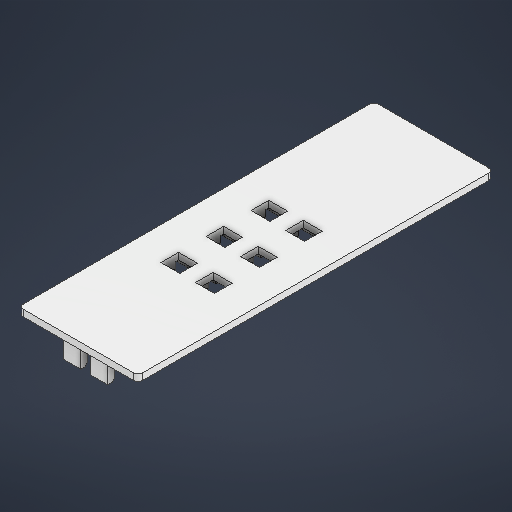
# Autodesk Inventor part: module-lid_switch
Saved by Autodesk Inventor 2025.4 (Build 294407000, 407)
## iProperties
Created: 2025-09-07
Part Number: module-lid_switch
Material: PC/ABS Plastic
Document SubType Name: Modeling
Designer: sam
Density: 1.1 g/cm^3
Appearance: Smooth - White
Author: sam
Autodesk Inventor part; units mm, degrees
ref_plane "YZ Plane" through (0, 0, 0) normal (1, 0, 0) x (0, 1, 0)
ref_plane "XZ Plane" through (0, 0, 0) normal (0, 1, 0) x (-1, 0, 0)
ref_plane "XY Plane" through (0, 0, 0) normal (0, 0, 1) x (1, 0, 0)
sketch "Sketch1" plane through (0, 0, 0) normal (0, 1, 0) x (-1, 0, 0)
  line L0 (-27.2, -81) -> (27.2, -81)
  line L1 (27.2, -81) -> (27.2, 81)
  line L2 (27.2, 81) -> (-27.2, 81)
  line L3 (-27.2, 81) -> (-27.2, -81)
  line L4 (-27.2, -81) -> (27.2, 81) construction
  line L5 (27.2, -81) -> (-27.2, 81) construction
  point P0 (0, 0)
  dimension "d0" = 54.4
  dimension "d1" = 162
  constraints: 12 end point, 2 midpoint, 2 parallel, 1 horizontal, 1 perpendicular
  measures "d0" distance of L2.end L1.end
  measures "d1" distance between parallel lines of L0 L2
extrude "Extrusion1" add sketch "Sketch1" along normal blind 3
sketch "Sketch2" plane through (0, 0, 0) normal (0, -1, 0) x (1, 0, 0)
  line L0 (24, 77.8) -> (-24, 77.8)
  line L1 (-24, 77.8) -> (-24, -77.8)
  line L2 (-24, -77.8) -> (24, -77.8)
  line L3 (24, -77.8) -> (24, 77.8)
  line L4 (24, 77.8) -> (-24, -77.8) construction
  line L5 (-24, 77.8) -> (24, -77.8) construction
  line L6 (-27.2, -81) -> (-27.2, 81) projected
  line L7 (27.2, -81) -> (-27.2, -81) projected
  point P0 (0, 0)
  dimension "d4" = 3.2
  dimension "d5" = 3.2
  constraints: 12 end point, 2 midpoint, 2 parallel, 1 horizontal, 1 perpendicular
  measures "d4" distance between parallel lines of L6 L1
  measures "d5" distance between parallel lines of L7 L2
extrude "Extrusion2" add sketch "Sketch2" along normal blind 3
fillet "Fillet1" radius 2 8 edges at (27.2, 1.5, 81) (24, -1.5, 77.8) (-24, -1.5, 77.8) (-27.2, 1.5, 81) (24, -1.5, -77.8) (27.2, 1.5, -81) (-27.2, 1.5, -81) (-24, -1.5, -77.8)
fillet "Fillet2" radius 0.5 8 edges at (-23.4142, -3, 77.2142) (-24, -3, 0) (-23.4142, -3, -77.2142) (0, -3, -77.8) (23.4142, -3, -77.2142) (24, -3, 0) (23.4142, -3, 77.2142) (0, -3, 77.8)
sketch "Sketch3" plane through (0, -3, 0) normal (0, -1, 0) x (1, 0, 0)
  line L0 (-22, 77.8) -> (22, 77.8) projected
  line L1 (-10.2, 77.8) -> (-2.14, 77.8)
  line L2 (-2.14, 77.8) -> (-2.14, 74.8)
  line L3 (-2.14, 74.8) -> (-10.2, 74.8)
  line L4 (-10.2, 74.8) -> (-10.2, 77.8)
  line L5 (-27.2, -79) -> (-27.2, 79) projected
  line L6 (2.14, 77.8) -> (10.2, 77.8)
  line L7 (10.2, 77.8) -> (10.2, 74.8)
  line L8 (10.2, 74.8) -> (2.14, 74.8)
  line L9 (2.14, 74.8) -> (2.14, 77.8)
  line L10 (27.2, 79) -> (27.2, -79) projected
  point P0 (0, 0)
  dimension "d10" = 8.06
  dimension "d11" = 3
  dimension "d12" = 17
  dimension "d13" = 8.06
  dimension "d14" = 3
  dimension "d15" = 17
  dimension "d17" = 0
  constraints: 16 end point, 4 parallel, 2 horizontal, 2 perpendicular, 1 point on line
  measures "d10" distance of L2.end L3.end
  measures "d11" distance of L1.end L2.end
  measures "d12" distance between parallel lines of L5 L4
  measures "d13" distance of L7.end L8.end
  measures "d14" distance of L6.end L7.end
  measures "d15" distance between parallel lines of L10 L7
  measures "d17" distance between parallel lines of L0 L6
extrude "Extrusion3" add sketch "Sketch3" along normal blind 10.8 from surface at -3
chamfer "Chamfer1" distance 1 angle 45 2 edges at (-6.17, -10.8, 74.8) (6.17, -10.8, 74.8)
sketch "Sketch5" plane through (0, 3, 0) normal (0, 1, 0) x (1, 0, 0)
  arc A0 (-25.2, 81) -> (-27.2, 79) centre (-25.2, 79) ccw projected
  line L0 (-27.2, 79) -> (-27.2, -79) projected
  arc A1 (-27.2, -79) -> (-25.2, -81) centre (-25.2, -79) ccw projected
  line L1 (-25.2, -81) -> (25.2, -81) projected
  arc A2 (25.2, -81) -> (27.2, -79) centre (25.2, -79) ccw projected
  line L2 (27.2, -79) -> (27.2, 79) projected
  arc A3 (27.2, 79) -> (25.2, 81) centre (25.2, 79) ccw projected
  line L3 (25.2, 81) -> (-25.2, 81) projected
  line L4 (-12.2, 18) -> (-3.6, 18)
  line L5 (-3.6, 18) -> (-3.6, 9.94)
  line L6 (-3.6, 9.94) -> (-12.2, 9.94)
  line L7 (-12.2, 9.94) -> (-12.2, 18)
  line L8 (12.2, 18) -> (3.6, 18)
  line L9 (3.6, 18) -> (3.6, 9.94)
  line L10 (3.6, 9.94) -> (12.2, 9.94)
  line L11 (12.2, 9.94) -> (12.2, 18)
  line L12 (-12.2, -2.56) -> (-3.6, -2.56)
  line L13 (-3.6, -2.56) -> (-3.6, -10.62)
  line L14 (-3.6, -10.62) -> (-12.2, -10.62)
  line L15 (-12.2, -10.62) -> (-12.2, -2.56)
  line L16 (12.2, -2.56) -> (3.6, -2.56)
  line L17 (3.6, -2.56) -> (3.6, -10.62)
  line L18 (3.6, -10.62) -> (12.2, -10.62)
  line L19 (12.2, -10.62) -> (12.2, -2.56)
  line L20 (-12.2, -23.12) -> (-3.6, -23.12)
  line L21 (-3.6, -23.12) -> (-3.6, -31.18)
  line L22 (-3.6, -31.18) -> (-12.2, -31.18)
  line L23 (-12.2, -31.18) -> (-12.2, -23.12)
  line L24 (12.2, -23.12) -> (3.6, -23.12)
  line L25 (3.6, -23.12) -> (3.6, -31.18)
  line L26 (3.6, -31.18) -> (12.2, -31.18)
  line L27 (12.2, -31.18) -> (12.2, -23.12)
  point P0 (0, 0)
  dimension "d35" = 8.6
  dimension "d36" = 8.06
  dimension "d37" = 63
  dimension "d38" = 15
  dimension "d39" = 8.6
  dimension "d40" = 63
  dimension "d41" = 15
  dimension "d42" = 8.06
  dimension "d45" = 8.6
  dimension "d46" = 8.06
  dimension "d47" = 8.6
  dimension "d48" = 8.06
  dimension "d49" = 8.6
  dimension "d50" = 8.06
  dimension "d51" = 8.6
  dimension "d52" = 8.06
  dimension "d57" = 15
  dimension "d58" = 15
  dimension "d59" = 15
  dimension "d60" = 15
  dimension "d61" = 12.5
  dimension "d62" = 12.5
  dimension "d63" = 12.5
  dimension "d64" = 12.5
  constraints: 48 end point, 12 parallel, 6 horizontal, 6 perpendicular
  measures "d35" distance of L5.end L6.end
  measures "d36" distance of L4.end L5.end
  measures "d37" distance between parallel lines of L3 L4
  measures "d38" distance between parallel lines of L0 L7
  measures "d39" distance of L10.end L9.end
  measures "d40" distance between parallel lines of L3 L8
  measures "d41" distance between parallel lines of L2 L11
  measures "d42" distance between parallel lines of L8 L10
  measures "d45" distance of L14.start L14.end
  measures "d46" distance of L13.start L14.start
  measures "d47" distance of L18.end L18.start
  measures "d48" distance between parallel lines of L16 L18
  measures "d49" distance of L22.start L22.end
  measures "d50" distance of L21.start L22.start
  measures "d51" distance of L26.end L26.start
  measures "d52" distance between parallel lines of L24 L26
  measures "d57" distance between parallel lines of L0 L15
  measures "d58" distance between parallel lines of L2 L19
  measures "d59" distance between parallel lines of L2 L27
  measures "d60" distance between parallel lines of L0 L23
  measures "d61" distance between parallel lines of L6 L12
  measures "d62" distance between parallel lines of L10 L16
  measures "d63" distance between parallel lines of L14 L20
  measures "d64" distance between parallel lines of L18 L24
extrude "Extrusion5" cut sketch "Sketch5" against normal through all contours L4 L5 L6 L7 | L11 L10 L9 L8 | L12 L13 L14 L15 | L19 L18 L17 L16 | L20 L21 L22 L23 | L27 L26 L25 L24
sketch "Sketch6" plane through (0, -3, 0) normal (0, -1, 0) x (1, 0, 0)
  line L0 (8.2, -17.6) -> (2.8, -17.6)
  line L1 (2.8, -17.6) -> (2.8, 32.4)
  line L2 (2.8, 32.4) -> (8.2, 32.4)
  line L3 (8.2, 32.4) -> (8.2, -17.6)
  line L4 (-8.2, 32.4) -> (-2.8, 32.4)
  line L5 (-2.8, 32.4) -> (-2.8, -17.6)
  line L6 (-2.8, -17.6) -> (-8.2, -17.6)
  line L7 (-8.2, -17.6) -> (-8.2, 32.4)
  line L8 (26, -16.6) -> (-26, -16.6)
  line L9 (-26, -16.6) -> (-26, -20)
  line L10 (-26, -20) -> (26, -20)
  line L11 (26, -20) -> (26, -16.6)
  line L12 (2.8, -17.6) -> (-2.8, -17.6)
  line L13 (26, 0.56) -> (-26, 0.56)
  line L14 (-26, 0.56) -> (-26, 3.96)
  line L15 (-26, 3.96) -> (26, 3.96)
  line L16 (26, 3.96) -> (26, 0.56)
  line L17 (26, 21.12) -> (-26, 21.12)
  line L18 (-26, 21.12) -> (-26, 24.52)
  line L19 (-26, 24.52) -> (26, 24.52)
  line L20 (26, 24.52) -> (26, 21.12)
  line L21 (25.2, -81) -> (-25.2, -81) projected
  line L22 (27.2, 79) -> (27.2, -79) projected
  point P0 (0, 0)
  point P1 (0, -17.6)
  point P2 (0, -20)
  point P3 (0, 0.56)
  point P4 (8.2, 0.56)
  point P5 (8.2, 3.96)
  point P6 (8.2, 21.12)
  point P7 (8.2, 24.52)
  point P8 (2.8, 24.52)
  point P9 (-2.8, 24.52)
  point P10 (-8.2, 24.52)
  point P11 (-8.2, 21.12)
  point P12 (-8.2, 3.96)
  point P13 (-8.2, 0.56)
  point P14 (-8.2, -16.6)
  point P15 (8.2, -16.6)
  point P16 (2.8, 3.96)
  point P17 (-2.8, 3.96)
  point P18 (-2.8, 21.12)
  point P19 (2.8, 21.12)
  point P20 (2.8, 0.56)
  point P21 (2.8, -16.6)
  point P22 (-2.8, -16.6)
  point P23 (-2.8, 0.56)
  dimension "d65" = 5.4
  dimension "d66" = 50
  dimension "d67" = 5.4
  dimension "d68" = 50
  dimension "d69" = 52
  dimension "d70" = 3.4
  dimension "d71" = 1
  dimension "d72" = 0
  dimension "d73" = 52
  dimension "d74" = 3.4
  dimension "d75" = 52
  dimension "d76" = 3.4
  dimension "d77" = 20.56
  dimension "d78" = 20.56
  dimension "d79" = 16.4
  dimension "d80" = 0
  dimension "d81" = 61
  dimension "d82" = 1.2
  constraints: 42 end point, 10 parallel, 5 horizontal, 5 perpendicular, 3 midpoint, 1 collinear, 1 point on line
  measures "d65" distance of L1.end L3.start
  measures "d66" distance of L0.end L1.end
  measures "d67" distance between parallel lines of L7 L5
  measures "d68" distance between parallel lines of L4 L6
  measures "d69" distance of L11.start L9.end
  measures "d70" distance of L9.end L9.start
  measures "d71" distance between parallel lines of L6 L8
  measures "d72" horizontal distance of point (0, -17.6) point (0, -20)
  measures "d73" distance of L14.end L16.start
  measures "d74" distance of L14.start L14.end
  measures "d75" distance of L19.start L20.start
  measures "d76" distance of L18.start L19.start
  measures "d77" distance between parallel lines of L15 L8
  measures "d78" distance between parallel lines of L19 L15
  measures "d79" distance between parallel lines of L7 L3
  measures "d80" horizontal distance of point (0, -17.6) point (0, 0.56)
  measures "d81" distance between parallel lines of L21 L10
  measures "d82" distance between parallel lines of L22 L11
extrude "Extrusion6" cut sketch "Sketch6" against normal blind 3 contours L3 L8 L11 L10 L9 L7 L6 L12 L0 | L0 L1 L8 L3 | L12 L5 L8 L1 | L8 L1 L13 L3 | L6 L7 L8 L5 | L13 L1 L15 L3 | L3 L15 L16 L13 | L13 L5 L15 L1 | L8 L7 L13 L5 | L15 L1 L17 L3 | L13 L7 L15 L5 | L17 L1 L19 L3 | L3 L19 L20 L17 | L17 L5 L19 L1 | L15 L7 L17 L5 | L13 L14 L15 L7 | L19 L1 L2 L3 | L17 L7 L19 L5 | L19 L7 L4 L5 | L17 L18 L19 L7
equation "\"d62\" = d61"
equation "\"d63\" = d61"
equation "\"d64\" = d63"
equation "\"d67\" = d65"
equation "\"d68\" = d66"
body "Solid1"
